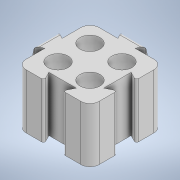
# Autodesk Inventor part: 4x11mmFlatBottom
Saved by Autodesk Inventor 2022.2 (Build 262287010, 287A)
## iProperties
Part Number: 4x11mmFlatBottom
Material: Generic
Document SubType Name: Modeling
Designer: yiunf
Appearance: Default
Author: yiunf
## iProperties of the stored document 4x11mm_3DPrint.ipt
Part Number: 4x11mm_3DPrint
Material: Generic
Document SubType Name: Modeling
Designer: yiunf
Appearance: Default
Author: yiunf
Autodesk Inventor part; units mm, degrees
ref_plane "YZ Plane" through (0, 0, 0) normal (1, 0, 0) x (0, 1, 0)
ref_plane "XZ Plane" through (0, 0, 0) normal (0, 1, 0) x (-1, 0, 0)
sketch "Sketch1" plane through (0, 0, 0) normal (0, 1, 0) x (-1, 0, 0)
  line L0 (-20, -20) -> (20, -20)
  line L1 (20, -20) -> (20, 20)
  line L2 (20, 20) -> (-20, 20)
  line L3 (-20, 20) -> (-20, -20)
  line L4 (-20, -20) -> (20, 20) construction
  line L5 (20, -20) -> (-20, 20) construction
  line L6 (20, 0) -> (25, 0)
  line L7 (25, 0) -> (25, 7.5)
  line L8 (20, 0) -> (20, 5)
  line L9 (20, 5) -> (25, 7.5)
  line L10 (25, 0) -> (25, -7.5)
  line L11 (20, 0) -> (20, -5)
  line L12 (20, -5) -> (25, -7.5)
  line L13 (0, -20) -> (5, -20)
  line L14 (0, -20) -> (-5, -20)
  line L15 (0, -20) -> (0, -25)
  line L16 (0, -25) -> (7.5, -25)
  line L17 (7.5, -25) -> (5, -20)
  line L18 (0, -25) -> (-7.5, -25)
  line L19 (-7.5, -25) -> (-5, -20)
  line L20 (-15, 0) -> (-15, -7.5)
  line L21 (-20, -5) -> (-15, -7.5)
  line L22 (-20, 0) -> (-15, 0)
  line L23 (-15, 0) -> (-15, 7.5)
  line L24 (-20, 5) -> (-15, 7.5)
  line L25 (-7.5, 15) -> (-5, 20)
  line L26 (0, 15) -> (-7.5, 15)
  line L27 (0, 20) -> (0, 15)
  line L28 (7.5, 15) -> (5, 20)
  line L29 (0, 15) -> (7.5, 15)
  line L30 (0, -24.75) -> (7.0955, -24.75)
  line L31 (7.0955, -24.75) -> (4.8455, -20.25)
  line L32 (4.8455, -20.25) -> (0, -20.25)
  line L33 (0, -24.75) -> (-7.0955, -24.75)
  line L34 (-7.0955, -24.75) -> (-4.8455, -20.25)
  line L35 (-4.8455, -20.25) -> (0, -20.25)
  line L36 (7.0955, -24.75) -> (4.7205, -20)
  line L37 (-7.0955, -24.75) -> (-4.7205, -20)
  line L38 (24.75, 0) -> (24.75, -7.0955)
  line L39 (24.75, -7.0955) -> (20.25, -4.8455)
  line L40 (20.25, -4.8455) -> (20.25, 0)
  line L41 (24.75, 0) -> (24.75, 7.0955)
  line L42 (24.75, 7.0955) -> (20.25, 4.8455)
  line L43 (20.25, 4.8455) -> (20.25, 0)
  line L44 (24.75, -7.0955) -> (20, -4.7205)
  line L45 (24.75, 7.0955) -> (20, 4.7205)
  line L46 (25, 0) -> (23.75, 0)
  line L47 (23.75, 0) -> (23.75, -6.875)
  line L48 (23.75, 0) -> (23.75, 6.875)
  line L49 (0, -25) -> (0, -23.75)
  line L50 (0, -23.75) -> (-6.875, -23.75)
  line L51 (0, -23.75) -> (6.875, -23.75)
  point P0 (0, 0)
  point P1 (-4.7205, -20)
  point P2 (4.7205, -20)
  point P3 (20, -4.7205)
  point P4 (20, 4.7205)
  point P5 (23.75, -6.5955)
  point P6 (23.75, 6.5955)
  point P7 (-6.5955, -23.75)
  point P8 (6.5955, -23.75)
  dimension "d0" = 40
  dimension "d1" = 40
  dimension "d2" = 5
  dimension "d3" = 7.5
  dimension "d4" = 5
  dimension "d5" = 7.5
  dimension "d6" = 5
  dimension "d7" = 5
  dimension "d8" = 5
  dimension "d9" = 5
  dimension "d10" = 7.5
  dimension "d11" = 7.5
  dimension "d14" = 40
  dimension "d21" = 40
  dimension "d43" = 0.25
  dimension "d44" = 0.25
  dimension "d45" = 0.25
  dimension "d46" = 0.25
  dimension "d56" = 1.25
  dimension "d57" = 1.25
  constraints: 104 end point, 21 point on line, 5 perpendicular, 4 midpoint, 3 horizontal, 3 parallel, 3 vertical, 30 other
  measures "d0" distance of L2.end L1.end
  measures "d1" distance of L1.end L0.end
  measures "d2" distance of L6.start L6.end
  measures "d3" distance of L6.end L7.end
  measures "d4" distance of L6.start L8.end
  measures "d5" distance of L6.end L10.end
  measures "d6" distance of L6.start L11.end
  measures "d7" distance of L13.start L13.end
  measures "d8" distance of L13.start L14.end
  measures "d9" distance of L13.start L15.end
  measures "d10" distance of L15.end L16.end
  measures "d11" distance of L15.end L18.end
  measures "d14" distance of L10.end L20.end
  measures "d21" distance of L18.end L25.start
  measures "d43" distance between parallel lines of L16 L30
  measures "d44" distance between parallel lines of L18 L33
  measures "d45" distance between parallel lines of L10 L38
  measures "d46" distance between parallel lines of L7 L41
  measures "d56" distance of L6.end L46.end
  measures "d57" distance of L15.end L49.end
extrude "Extrusion1" add sketch "Sketch1" along normal blind 30 contours L3 L21 L20 L23 L24 L2 L25 L26 L29 L28 L1 L0 | L0 L15 L35 L37 | L0 L36 L32 L15 | L35 L15 L50 L34 | L32 L31 L51 L15 | L1 L6 L40 L44 | L1 L45 L43 L6 | L40 L6 L47 L39 | L43 L42 L48 L6
sketch "Sketch2" plane through (0, 30, 0) normal (0, 1, 0) x (1, 0, 0)
  line L0 (-4.7205, 20) -> (-20, 20) projected
  line L1 (-20, 20) -> (0, 20)
  line L2 (0, 20) -> (0, 0)
  circle A0 centre (-10, 10) radius 5.5
  circle A1 centre (7.5, 10) radius 5.5
  circle A2 centre (-10, -7.5) radius 5.5
  circle A3 centre (7.5, -7.5) radius 5.5
  point P0 (-5, 20)
  dimension "d30" = 11
  dimension "d33" = 17.5
  dimension "d36" = 17.5
  constraints: 4 centre point, 4 end point, 2 horizontal, 1 perpendicular, 1 vertical, 6 other
  measures "d30" diameter of A0
  measures "d33" distance of A0.centre A1.centre
  measures "d36" distance of A0.centre A2.centre
extrude "Extrusion2" cut sketch "Sketch2" against normal blind 25
fillet "Fillet1" radius 1 4 edges at (20, 15, -5) (20, 15, 5) (5, 15, 20) (-5, 15, 20)
fillet "Fillet2" radius 5 4 edges at (20, 15, -20) (20, 15, 20) (-20, 15, 20) (-20, 15, -20)
ref_plane "Work Plane1" through (6.5955, 0, -23.75) normal (-1, 0, 0) x (0, 1, 0)
sketch "Sketch3" plane through (6.5955, 0, -23.75) normal (-1, 0, 0) x (0, 1, 0)
  line L0 (0, -3.75) -> (30, -3.75) projected
  line L1 (15, -3.75) -> (15, 2)
  line L2 (0, 0) -> (5, 0)
  line L3 (15, 2) -> (15, -0.25)
  line L4 (15, 2) -> (15, 0.875)
  line L5 (30, -3.75) -> (30, 0) projected
  line L6 (25, 0) -> (30, 0)
  line L7 (0, 0) -> (30, 0) projected
  arc A0 (30, 0) -> (0, 0) centre (15, -55.25) ccw
  line L8 (15, 2) -> (15, 1)
  arc A1 (25, 0) -> (5, 0) centre (15, -49.5) ccw
  point P0 (0, -23.75)
  dimension "d48" = 5.75
  dimension "d55" = 5
  dimension "d60" = 1
  dimension "d61" = 5
  constraints: 12 end point, 6 point on circle, 2 centre point, 2 horizontal, 2 midpoint, 1 point on line, 1 vertical, 1 other
  measures "d48" distance of L1.start L1.end
  measures "d55" distance of L2.start L2.end
  measures "d60" distance of L1.end L8.end
  measures "d61" distance of L6.start L5.end
extrude "Extrusion3" add sketch "Sketch3" along normal blind 13.191 contours L6 A1 L1 A0 | L1 A1 L2 A0
pattern_circular "Circular Pattern1" count 2 over 90 about axis through (0, 30, 0) along (0, 1, 0) of "Extrusion3"
fillet "Fillet3" radius 2 4 edges at (0, 30, -23.75) (0, 0, -23.75) (-23.75, 30, 0) (-23.75, 0, 0)
sketch "Sketch5" plane through (-6.5955, 0, -23.75) normal (-1, 0, 0) x (0, 0, 1)
  point P0 (23.75, 0)
body "Solid1"
